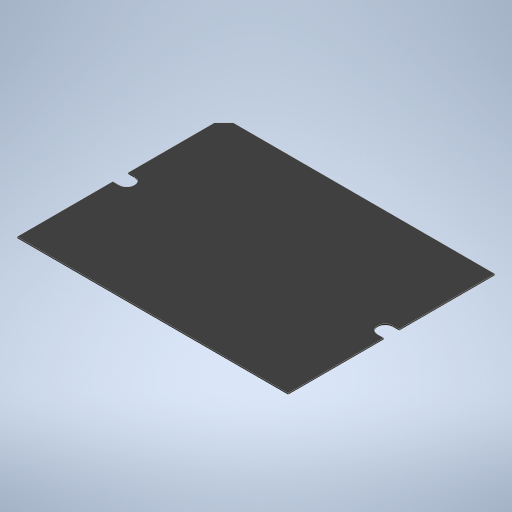
# Autodesk Inventor part: Thermal Pad
Saved by Autodesk Inventor 2023 (Build 270158000, 158)
## iProperties
Created: 2023-03-13
Part Number: Thermal Pad
Material: Rubber, Silicone
Document SubType Name: Modeling
Designer: Caleb
Density: 1.25 g/cm^3
Appearance: Rubber - Black
Author: Caleb
Autodesk Inventor part; units mm, degrees
ref_plane "YZ Plane" through (0, 0, 0) normal (1, 0, 0) x (0, 1, 0)
ref_plane "XZ Plane" through (0, 0, 0) normal (0, 1, 0) x (-1, 0, 0)
ref_plane "XY Plane" through (0, 0, 0) normal (0, 0, 1) x (1, 0, 0)
sketch "Sketch1" plane through (0, 0, 0) normal (0, 1, 0) x (-1, 0, 0)
  line L0 (-28.25, -21.55) -> (28.25, -21.55)
  line L1 (28.25, -21.55) -> (28.25, 21.55)
  line L2 (28.25, 21.55) -> (-28.25, 21.55)
  line L3 (-28.25, 21.55) -> (-28.25, -21.55)
  line L4 (-28.25, -21.55) -> (28.25, 21.55) construction
  line L5 (28.25, -21.55) -> (-28.25, 21.55) construction
  point P0 (0, 0)
  dimension "d0" = 43.1
  dimension "d1" = 56.5
  constraints: 12 end point, 2 midpoint, 2 parallel, 1 horizontal, 1 perpendicular
  measures "d0" distance of L0.end L1.end
  measures "d1" distance of L1.end L2.end
extrude "Extrusion1" add sketch "Sketch1" along normal blind 0.25
chamfer "Chamfer1" distance 2 angle 45 1 edges at (-28.25, 0.125, -21.55)
sketch "Sketch2" plane through (0, 0.25, 0) normal (0, 1, 0) x (1, 0, 0)
  line L0 (0, 21.55) -> (0, -21.55) construction
  line L1 (-28.25, 19.55) -> (-28.25, -21.55) projected
  line L2 (-28.25, -21.55) -> (28.25, -21.55) projected
  line L3 (28.25, 21.55) -> (-26.25, 21.55) projected
  line L4 (-28.25, 0) -> (28.25, 0) construction
  line L5 (28.25, -21.55) -> (28.25, 21.55) construction
  line L6 (-28.25, 1.6) -> (-26.95, 1.6)
  line L7 (-28.25, -1.6) -> (-26.95, -1.6)
  line L8 (-28.25, 19.55) -> (-28.25, -21.55) construction
  arc A0 (-26.95, -1.6) -> (-26.95, 1.6) centre (-26.95, 0) ccw
  line L9 (28.25, 19.55) -> (28.25, -21.55)
  line L10 (28.25, 0) -> (-28.25, 0) construction
  line L11 (28.25, 1.6) -> (26.95, 1.6)
  line L12 (28.25, -1.6) -> (26.95, -1.6)
  line L13 (28.25, 19.55) -> (28.25, -21.55) construction
  arc A1 (26.95, 1.6) -> (26.95, -1.6) centre (26.95, 0) ccw
  point P0 (0, 0)
  dimension "d14" = 3.2
  dimension "d15" = 1.3
  dimension "d16" = 1.3
  dimension "d17" = 3.2
  dimension "d18" = 1.6
  constraints: 18 end point, 8 symmetric about line, 7 point on line, 4 point on circle, 3 midpoint, 2 centre point, 2 parallel, 1 perpendicular, 1 vertical, 1 other
  measures "d14" diameter of L6 L4
  measures "d15" distance of L6.start L6.end
  measures "d16" distance of L7.start L7.end
  measures "d17" diameter of L7 L4
  measures "d18" radius of A0
extrude "Extrusion2" cut sketch "Sketch2" against normal through all
equation "\"d16\" = d15"
equation "\"d17\" = d14"
equation "\"d18\" = 0.5 * d14"
body "Solid1"
